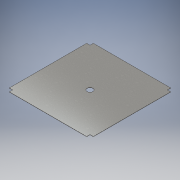
# Autodesk Inventor part: FrameSheetLaserViewport
Saved by Autodesk Inventor 2016 (Build 200138000, 138)
## iProperties
Created: 2015-08-02
Part Number: FrameSheetLaserViewport
Material: Steel, Galvanized
Document SubType Name: Sheet Metal
Designer: myhome
Density: 7.85 g/cm^3
Sheet Metal Rule: Default_mm
Appearance: Galvanized
Author: myhome
Autodesk Inventor part; units mm, degrees
ref_plane "YZ Plane" through (0, 0, 0) normal (1, 0, 0) x (0, 1, 0)
ref_plane "XZ Plane" through (0, 0, 0) normal (0, 1, 0) x (-1, 0, 0)
ref_plane "XY Plane" through (0, 0, 0) normal (0, 0, 1) x (1, 0, 0)
sketch "Sketch4" plane through (0, 0, 0) normal (0, 0, 1) x (1, 0, 0)
  line L0 (0, 0) -> (500, 0)
  line L1 (500, 0) -> (500, 500)
  line L2 (500, 500) -> (0, 500)
  line L3 (0, 500) -> (0, 0)
  dimension "d9" = 500
  dimension "d10" = 500
  measures "d9" distance of L1.end L2.end
  measures "d10" distance of L0.end L1.end
extrude "Plate2" add sketch "Sketch4" along normal blind 1.214
sketch "Sketch7" plane through (0, 0, 0) normal (0, 0, 1) x (1, 0, 0)
  line L0 (0, 0) -> (20, 0)
  line L1 (20, 0) -> (20, 20)
  line L2 (20, 20) -> (0, 20)
  line L3 (0, 20) -> (0, 0)
  dimension "d16" = 20
  dimension "d17" = 20
  constraints: 8 end point, 2 parallel, 1 horizontal, 1 perpendicular
  measures "d16" distance of L2.end L1.end
  measures "d17" distance of L0.end L1.end
extrude "Cut4" cut sketch "Sketch7" along normal blind 1.214
sketch "Sketch8" plane through (0, 0, 0) normal (0, 0, 1) x (1, 0, 0)
  line L0 (500, 0) -> (500, 500) projected
  line L1 (500, 0) -> (480, 0)
  line L2 (480, 0) -> (480, 20)
  line L3 (480, 20) -> (500, 20)
  line L4 (500, 20) -> (500, 0)
  line L5 (500, 500) -> (480, 500)
  line L6 (480, 500) -> (480, 480)
  line L7 (480, 480) -> (500, 480)
  line L8 (500, 480) -> (500, 500)
  line L9 (500, 500) -> (0, 500) projected
  line L10 (0, 500) -> (20, 500)
  line L11 (20, 500) -> (20, 480)
  line L12 (20, 480) -> (0, 480)
  line L13 (0, 480) -> (0, 500)
  point P0 (0, 0)
  dimension "d20" = 20
  dimension "d21" = 20
  dimension "d22" = 20
  dimension "d23" = 20
  dimension "d24" = 20
  dimension "d25" = 20
  constraints: 24 end point, 6 parallel, 3 horizontal, 3 perpendicular
  measures "d20" distance of L2.end L3.end
  measures "d21" distance of L1.end L2.end
  measures "d22" distance of L7.end L6.end
  measures "d23" distance of L5.end L6.end
  measures "d24" distance of L11.end L12.end
  measures "d25" distance of L10.end L11.end
extrude "Cut5" cut sketch "Sketch8" along normal blind 1.214
sketch "Sketch10" plane through (0, 0, 0) normal (0, 0, 1) x (1, 0, 0)
  line L0 (0, 0) -> (250, 0)
  line L1 (480, 0) -> (20, 0) projected
  line L2 (0, 0) -> (0, 250)
  line L3 (0, 250) -> (250, 250)
  circle A0 centre (250, 250) radius 17.5
  dimension "d31" = 250
  dimension "d32" = 250
  dimension "d33" = 35
  constraints: 6 end point, 1 centre point, 1 coincident, 1 midpoint, 1 perpendicular, 1 vertical
  measures "d31" distance of L0.start L2.end
  measures "d32" distance of L2.end L3.end
  measures "d33" diameter of A0
extrude "Cut6" cut sketch "Sketch10" along normal up to next
equation "\"d18\" = Thickness"
equation "\"d26\" = Thickness"
equation "\"d34\" = Thickness"
equation "\"BendRadius\" = Thickness"
equation "\"BendReliefWidth\" = Thickness"
equation "\"BendReliefDepth\" = 0.5 * Thickness"
equation "\"CornerReliefSize\" = 4 * Thickness"
equation "\"MinimumRemnant\" = 2 * Thickness"
equation "\"TransitionRadius\" = BendRadius"
equation "\"JacobiRadiusSize\" = BendRadius"
equation "\"GapSize\" = Thickness"
equation "\"d2\" = BendRadius"
equation "\"d11\" = BendRadius"
equation "\"Thickness\" = 1.214"
body "Solid2"
